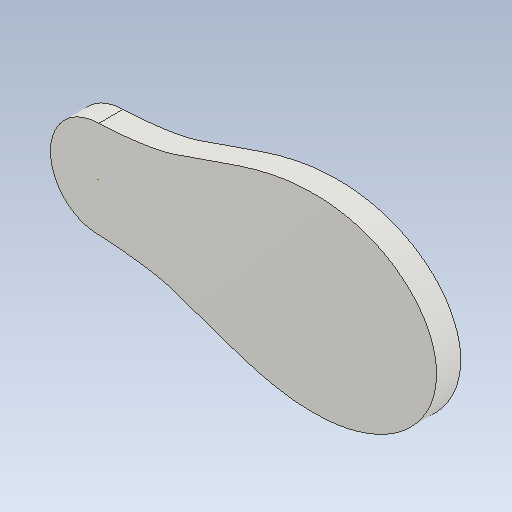
# Autodesk Inventor part: Disc Cam
Saved by Autodesk Inventor 2020.2 (Build 242310000, 310)
## iProperties
Created: 2020-01-19
Part Number: Disc Cam
Material: Stainless Steel, Austenitic
Document SubType Name: Modeling
Designer: robst
Manufacturer: Standard
Standards Organization: Custom
Density: 1 g/cm^3
Appearance: Steel
CustomPartVersion: 1
Author: robst
Autodesk Inventor part; units mm, degrees
ref_plane "YZ Plane" through (0, 0, 0) normal (1, 0, 0) x (0, 1, 0)
ref_plane "XZ Plane" through (0, 0, 0) normal (0, 1, 0) x (-1, 0, 0)
ref_plane "XY Plane" through (0, 0, 0) normal (0, 0, 1) x (1, 0, 0)
sketch "Main Sketch" plane through (0, 0, 0) normal (0, 0, 1) x (1, 0, 0)
  spline S0 degree 5 poles (0, 25.4) (2.5068, 25.4931) (9.5937, 25.8216) (34.8963, 28.1564) (41.5022, 32.3932) (61.3156, 38.3245) (73.3405, 43.1303) (87.0629, 47.0563) (99.9877, 49.5752) (113.2442, 50.4728) (126.2764, 49.526) (138.8345, 46.6154) (150.3187, 41.7811) (160.2305, 35.2501) (168.149, 27.3952) (173.8405, 18.6526) (177.2328, 9.423) (178.3549, 0) (177.2328, -9.423) (173.8405, -18.6526) (168.1489, -27.3952) (160.2308, -35.2501) (150.318, -41.781) (138.8363, -46.6156) (126.2719, -49.5255) (113.2549, -50.4742) (99.9621, -49.5719) (87.1249, -47.0644) (73.1808, -43.1095) (61.5404, -38.2984) (41.8653, -32.701) (37.8091, -28.6704) (1.2124, -24.8752) (-0.1512, -25.6423) (-4.5554, -25.1084) (-7.6308, -24.3085) (-10.3713, -23.2658) (-12.7298, -22.0583) (-14.9729, -20.6051) (-17.0416, -18.9279) (-18.9281, -17.0425) (-20.6053, -14.9708) (-22.0575, -12.7349) (-23.2677, -10.3595) (-24.2232, -7.8706) (-24.9132, -5.2955) (-25.3302, -2.6623) (-25.4697, 0) (-25.3302, 2.6623) (-24.9131, 5.2955) (-24.2232, 7.8706) (-23.2676, 10.3595) (-22.0577, 12.7348) (-20.6048, 14.9708) (-18.9292, 17.0424) (-17.0391, 18.9282) (-14.9789, 20.6044) (-12.7159, 22.06) (-10.4035, 23.2618) (-7.8738, 24.1979) (-5.6183, 24.8588) (-2.9486, 25.2794) (-1.9297, 25.3364) (-0.863, 25.368) (0, 25.4) knots 0 0 0 0 0 0 0.035705 0.057661 0.08417 0.108857 0.132321 0.155218 0.177924 0.200525 0.222925 0.24495 0.266428 0.287249 0.30741 0.327033 0.346355 0.365676 0.3853 0.40546 0.426281 0.447759 0.469784 0.492184 0.514786 0.537492 0.560389 0.583852 0.608539 0.635048 0.659052 0.680389 0.698652 0.713195 0.723438 0.733681 0.743924 0.754167 0.76441 0.774653 0.784896 0.795139 0.805383 0.815626 0.825869 0.836112 0.846355 0.856598 0.866841 0.877084 0.887327 0.89757 0.907813 0.918056 0.928299 0.938542 0.948785 0.959028 0.969271 0.979514 0.987708 1 1 1 1 1 1
  point P0 (45.8011, 33.2758)
  point P1 (61.5045, 38.701)
  point P2 (74.8325, 43.2834)
  point P3 (87.474, 46.8499)
  point P4 (100.2409, 49.197)
  point P5 (113.3047, 50.0127)
  point P6 (126.4072, 48.9959)
  point P7 (139.0282, 45.9824)
  point P8 (150.5429, 41.0236)
  point P9 (160.3712, 34.3971)
  point P10 (168.1022, 26.5461)
  point P11 (173.5557, 17.9579)
  point P12 (176.7528, 9.0313)
  point P13 (177.8, 0)
  point P14 (176.7528, -9.0313)
  point P15 (173.5557, -17.9579)
  point P16 (168.1022, -26.5461)
  point P17 (160.3712, -34.3971)
  point P18 (150.5429, -41.0236)
  point P19 (139.0282, -45.9824)
  point P20 (126.4072, -48.9959)
  point P21 (113.3047, -50.0127)
  point P22 (100.2409, -49.197)
  point P23 (87.474, -46.8499)
  point P24 (74.8325, -43.2834)
  point P25 (61.5045, -38.701)
  point P26 (45.8011, -33.2758)
  point P27 (25.4096, -27.9142)
  point P28 (0, -25.4)
  point P29 (-2.655, -25.2609)
  point P30 (-5.281, -24.8449)
  point P31 (-7.849, -24.1568)
  point P32 (-10.3311, -23.2041)
  point P33 (-12.7, -21.997)
  point P34 (-14.9297, -20.549)
  point P35 (-16.9959, -18.8759)
  point P36 (-18.8759, -16.9959)
  point P37 (-20.549, -14.9297)
  point P38 (-21.997, -12.7)
  point P39 (-23.2041, -10.3311)
  point P40 (-24.1568, -7.849)
  point P41 (-24.8449, -5.281)
  point P42 (-25.2609, -2.655)
  point P43 (-25.4, 0)
  point P44 (-25.2609, 2.655)
  point P45 (-24.8449, 5.281)
  point P46 (-24.1568, 7.849)
  point P47 (-23.2041, 10.3311)
  point P48 (-21.997, 12.7)
  point P49 (-20.549, 14.9297)
  point P50 (-18.8759, 16.9959)
  point P51 (-16.9959, 18.8759)
  point P52 (-14.9297, 20.549)
  point P53 (-12.7, 21.997)
  point P54 (-10.3311, 23.2041)
  point P55 (-7.849, 24.1568)
  point P56 (-5.281, 24.8449)
  point P57 (-2.655, 25.2609)
  constraints: 60 other
extrude "Cam" add sketch "Main Sketch" along normal blind 12.7
body "Solid1"
